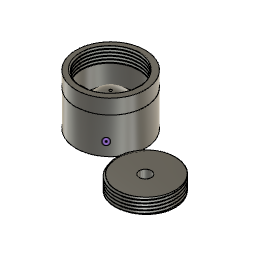
v5 (Autodesk Fusion 360 design; units mm, degrees)
Autodesk Fusion 360 part; units mm, degrees
note: some values were not read from the file. Set by a fixed rule: which face or edge a step refers to.
sketch "Sketch1" plane through (0, 0, 0) normal (0, 0, 1) x (1, 0, 0)
sketch "Sketch2" plane through (0, 0, 0) normal (0, 0, 1) x (1, 0, 0)
  circle A0 centre (0, 0) radius 10.5
  dimension "d3" = 21
  constraint coincident A0.centre origin
  measures "d3" diameter of A0
form "Form1" [no effect]
sketch "Sketch3" plane through (0, 0, 0) normal (0, 1, 0) x (1, 0, 0)
  circle A0 centre (0, 0) radius 11.5
  circle A1 centre (0, 0) radius 7.5
  circle A2 centre (0, 0) radius 10.5
  dimension "d7" = 23
  dimension "d8" = 15
  dimension "d9" = 21
  constraint coincident A0.centre A1.centre
  constraint concentric A0 A2
  measures "d7" diameter of A0
  measures "d8" diameter of A1
  measures "d9" diameter of A2
sketch "Sketch4" plane through (0, 0, 0) normal (0, 1, 0) x (1, 0, 0)
  line L0 (7, -0.5) -> (11, -0.5)
  line L1 (11, -0.5) -> (11, 0.5)
  line L2 (11, 0.5) -> (7, 0.5)
  line L3 (7, 0.5) -> (7, -0.5)
  line L4 (0.5, -7) -> (-0.5, -7)
  line L5 (-0.5, -7) -> (-0.5, -11)
  line L6 (-0.5, -11) -> (0.5, -11)
  line L7 (0.5, -11) -> (0.5, -7)
  line L8 (-7, 0.5) -> (-11, 0.5)
  line L9 (-11, 0.5) -> (-11, -0.5)
  line L10 (-11, -0.5) -> (-7, -0.5)
  line L11 (-7, -0.5) -> (-7, 0.5)
  line L12 (-0.5, 7) -> (0.5, 7)
  line L13 (0.5, 7) -> (0.5, 11)
  line L14 (0.5, 11) -> (-0.5, 11)
  line L15 (-0.5, 11) -> (-0.5, 7)
  constraint horizontal L0
  constraint vertical L1
  constraint horizontal L2
  constraint vertical L3
  constraint horizontal L4
  constraint vertical L5
  constraint horizontal L6
  constraint vertical L7
  constraint horizontal L8
  constraint vertical L9
  constraint horizontal L10
  constraint vertical L11
  constraint horizontal L12
  constraint vertical L13
  constraint horizontal L14
  constraint vertical L15
extrude "Extrude2" add sketch "Sketch3" along normal blind 20 and the other way blind 2 makes body 1 at (11.4857, 13.3333, 0.5732) makes body 2 at (7.4907, 13.3333, 0.3738)
extrude "Extrude3" add sketch "Sketch4" along normal blind 20 bodies 1 2
sketch "Sketch5" plane through (0, 0, 0) normal (0, 0, 1) x (1, 0, 0)
sketch "Sketch6" plane through (0, 0, 0) normal (0, 1, 0) x (1, 0, 0)
extrude "Extrude4" cut 14 faces at (-10.8871, 20, 2.3801) (-0.0556, 20, -10.8329) (-10.8329, 20, -0.0556) (-0.0556, 20, 10.8329) (10.8329, 20, 0.0556) (-0.3889, 20, -8.4898) (-8.4898, 20, -0.3889) (0.3889, 20, 8.4898) (8.4898, 20, -0.3889) (0.0556, 20, -7.166) (-7.166, 20, -0.0556) (0.0556, 20, 7.166) (7.166, 20, -0.0556) (-2, 20, -0.1667) along direction (0, -1, 0) blind 15 on bodies 1 bodies 1
sketch "Sketch7" plane through (0, 0, 0) normal (0, 1, 0) x (1, 0, 0)
  circle A0 centre (65, 0) radius 11.5
  circle A1 centre (65, 0) radius 7.5
  circle A2 centre (65, 0) radius 10.5
  dimension "d18" = 23
  dimension "d19" = 15
  dimension "d20" = 21
  constraint concentric A0 A1
  constraint concentric A0 A2
  measures "d18" diameter of A0
  measures "d19" diameter of A1
  measures "d20" diameter of A2
extrude "Extrude5" add sketch "Sketch7" along normal blind 5 separate body makes body 3 at (72.4907, 3.3333, 0.3738) makes body 4 at (76.4857, 3.3333, 0.5732)
fillet "Fillet1" radius 7.5 1 faces at (62.7476, 5, -1.0847) on bodies 3
combine "Combine1" operation add target body 3 tool bodies 4 makes body 5 at (76.4857, 3.3333, 0.5732)
combine "Combine2" operation add target body 1 tool bodies 3 makes body 6 at (71.9525, 0.9408, 1.4055)
move_body "Move2" bodies 5 6 to x (1, 0, 0) y (0, 1, 0) z (0, 0, 1) at (-65, 5, 0)
combine "Combine3" operation add target body 1 tool bodies 5
sketch "Sketch8" plane through (0, 0, 0) normal (0, 1, 0) x (1, 0, 0)
  circle A0 centre (70, 0) radius 11.5
  dimension "d25" = 23
  measures "d25" diameter of A0
move_face "OffsetFaces1" offset -1 1 faces at (6.9276, 5.9894, -1.4004) on bodies 6
extrude "Extrude7" add 1 faces at (11.1239, 10, 0.5713) along direction (0, -1, 0) blind 5 on bodies 1 bodies 1
sketch "Sketch9" plane through (0, 0, 0) normal (0, 1, 0) x (1, 0, 0)
  circle A0 centre (30, 0) radius 10.5
  dimension "d34" = 21
  measures "d34" diameter of A0
extrude "Extrude8" add sketch "Sketch9" along normal blind 5 separate body makes body 7
hole "Hole2" at (29.9465, 5, -0.108) direction (0, -1, 0) diameter 3.5 depth 5 tip angle 180 counterbore diameter 3.6 counterbore depth 1 bodies 7
sketch "Sketch10" plane through (0, 0, 0) normal (0, 1, 0) x (1, 0, 0)
sketch "Sketch11" plane through (0, 0, 0) normal (0, 1, 0) x (1, 0, 0)
  circle A0 centre (-25, 0) radius 11.5
  dimension "d43" = 23
  measures "d43" diameter of A0
extrude "Extrude9" add sketch "Sketch11" along normal blind 5 separate body makes body 8
hole "Hole3" at (-25, 5, 0) direction (0, -1, 0) diameter 21 depth 5 tip angle 180 counterbore diameter 21 counterbore depth 1 bodies 8
thread "Thread5" "ISO Metric profile 20.0 M20x1 6g" major diameter 19.884 minor diameter 18.7405 pitch 1 angle 60 resizes the face on face at (40.4869, 3.3333, 0.5234) on bodies 7
thread "Thread6" "ISO Metric profile 20.0 M20x1 6H" major diameter 20.152 minor diameter 19.035 pitch 1 angle 60 resizes the face on face at (-23.9545, 1.6667, 10.4478) on bodies 8
move_body "Move4" bodies 8 to x (1, 0, 0) y (0, 1, 0) z (0, 0, 1) at (24.8884, 30.8859, 0)
move_body "Move5" bodies 8 to x (1, 0, 0) y (0, 1, 0) z (0, 0, 1) at (0.1, -21, 0)
combine "Combine5" operation add target body 1 tool bodies 8 6
thread "Thread7" "ISO Metric profile 20.0 M20x1 6H" major diameter 20.152 minor diameter 19.035 pitch 1 angle 60 resizes the face on face at (0.4628, 13.2192, 9.5057) on bodies 1
move_body "Move6" bodies 7 to x (1, 0, 0) y (0, 0, 1) z (0, -1, 0) at (0, -9.942, -9.942)
move_body "Move7" bodies 1 to x (1, 0, 0) y (0, 0, 1) z (0, -1, 0) at (0, 2.5, -8.5)
move_body "Move8" bodies 1 to x (1, 0, 0) y (0, 1, 0) z (0, 0, 1) at (6, 0, 0.5)
copy_body "Body->Comp1" bodies 7 removing the originals makes body 9 in component "Component"
copy_body "Body->Comp2" bodies 1 removing the originals makes body 10 in component "Component'"
thread "Thread1" "ISO Metric profile 20.0 M20x1 6H" major diameter 20.152 minor diameter 19.035 pitch 1 angle 60 modelled right hand crest width 0.2719 on face at (6.4628, -7.0057, 5.2192) crest through (5.9884, -7.0175, 6.6359) on bodies 10 in component "Component'"
thread "Thread1'" "ISO Metric profile 20.0 M20x1 6g" major diameter 19.884 minor diameter 18.7405 pitch 1 angle 60 modelled right hand crest width 0.1426 on face at (39.9296, -9.4464, -8.2753) crest through (39.942, -9.942, -10.192) on bodies 9 in component "Component"
move_body "Move1" bodies 9 to x (1, 0, 0) y (0, 1, 0) z (0, 0, 1) at (-19, 12, 0) in component "Component"
move_body "Move1'" bodies 10 to x (1, 0, 0) y (0, 1, 0) z (0, 0, 1) at (-19, 12, 0) in component "Component'"
move_face "OffsetFaces1'" offset -0.5 2 faces at (11.1257, 0.375, -5.6087) (11.1207, 0.4247, -8.6087) on bodies 9 in component "Component"
delete_face "DeleteFace1" 1 faces at (11.0587, -0.0812, -7.2753) on bodies 9 in component "Component"
delete_face "DeleteFace2" 1 faces at (11.1755, -0.1226, -5.2753) on bodies 9 in component "Component"
hole "Hole1" at (11, 2.058, -4.942) direction (0, 0, -1) diameter 4 depth 5 tip angle 180 bodies 9 in component "Component"
thread "Thread4" [suppressed]
combine "Combine4" [suppressed]
thread "Thread2" [suppressed]
thread "Thread3" [suppressed]
thread "Thread1''" [suppressed]
component "Component" placed x (1, 0, 0) y (0, 1, 0) z (0, 0, 1) at (0, 0, 0)
component "Component'" placed x (1, 0, 0) y (0, 1, 0) z (0, 0, 1) at (0, 0, 0)
